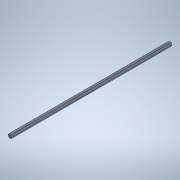
# Autodesk Inventor part: Intake hex
Saved by Autodesk Inventor 2022 (Build 260153000, 153)
## iProperties
Created: 2023-01-13
Part Number: Intake hex
Material: Aluminum 6061
Document SubType Name: Modeling
Designer: s135320
Mass: 192.018 g
Surface Area: 226.541 cm^2
Volume: 71.1179 cm^3
Density: 2.7 g/cm^3
Appearance: Aluminum - Flat
Author: s135320
Autodesk Inventor part; units mm, degrees
ref_plane "YZ Plane" through (0, 0, 0) normal (1, 0, 0) x (0, 1, 0)
ref_plane "XZ Plane" through (0, 0, 0) normal (0, 1, 0) x (-1, 0, 0)
ref_plane "XY Plane" through (0, 0, 0) normal (0, 0, 1) x (1, 0, 0)
sketch "Sketch1" plane through (0, 0, 0) normal (0, 0, 1) x (1, 0, 0)
  line L0 (7.3406, 0) -> (3.6703, -6.3571)
  line L1 (3.6703, -6.3571) -> (-3.6703, -6.3571)
  line L2 (-3.6703, -6.3571) -> (-7.3406, 0)
  line L3 (-7.3406, 0) -> (-3.6703, 6.3571)
  line L4 (-3.6703, 6.3571) -> (3.6703, 6.3571)
  line L5 (3.6703, 6.3571) -> (7.3406, 0)
  point P0 (0, 0)
  point P1 (0, 0)
  dimension "d0" = 7.3406
  constraints: 12 end point, 1 coincident, 13 other
  measures "d0" distance of L3.end L4.end
extrude "Extrusion1" add sketch "Sketch1" along normal blind 571.5
body "Solid1"
